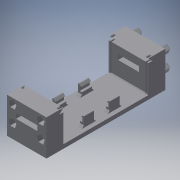
# Autodesk Inventor part: updated token 18mm
Saved by Autodesk Inventor 2018 (Build 220112000, 112)
## iProperties
Created: 2020-11-10
Part Number: updated token 18mm
Material: Generic
Document SubType Name: Modeling
Designer: Olivi
Density: 1 g/cm^3
Appearance: Default
Author: Olivi
Autodesk Inventor part; units mm, degrees
ref_plane "YZ Plane" through (0, 0, 0) normal (1, 0, 0) x (0, 1, 0)
ref_plane "XZ Plane" through (0, 0, 0) normal (0, 1, 0) x (-1, 0, 0)
ref_plane "XY Plane" through (0, 0, 0) normal (0, 0, 1) x (1, 0, 0)
sketch "Sketch1" plane through (0, 0, 0) normal (0, 0, 1) x (1, 0, 0)
  line L0 (0, 0) -> (20, 0)
  line L1 (20, 0) -> (20, 50)
  line L2 (20, 50) -> (0, 50)
  line L3 (0, 50) -> (0, 0)
  dimension "d0" = 20
  dimension "d1" = 50
  constraints: 8 end point, 2 parallel, 1 horizontal, 1 perpendicular
  measures "d0" distance of L2.end L1.end
  measures "d1" distance of L1.end L0.end
extrude "Extrusion1" add sketch "Sketch1" along normal blind 2
sketch "Sketch8" plane through (0, 0, 2) normal (0, 0, 1) x (1, 0, 0)
  line L0 (0, 0) -> (20, 0) projected
  line L1 (20, 0) -> (20, 50) projected
  line L2 (0, 0) -> (20, 0)
  line L3 (20, 0) -> (20, 8.5)
  line L4 (20, 8.5) -> (0, 8.5)
  line L5 (0, 8.5) -> (0, 0)
  dimension "d39" = 8.5
  constraints: 8 end point, 2 parallel, 1 horizontal, 1 perpendicular, 1 point on line
  measures "d39" distance of L3.end L2.end
extrude "Extrusion8" add sketch "Sketch8" along normal blind 16
sketch "Sketch9" plane through (0, 0, 0) normal (0, -1, 0) x (1, 0, 0)
  line L0 (20, 0) -> (20, 18) projected
  line L1 (0, 18) -> (20, 18) projected
  line L2 (0, 0) -> (0, 18) projected
  line L3 (4.67, 12.27) -> (15.33, 12.27)
  line L4 (15.33, 12.27) -> (15.33, 9.73)
  line L5 (15.33, 9.73) -> (4.67, 9.73)
  line L6 (4.67, 9.73) -> (4.67, 12.27)
  dimension "d42" = 4.67
  dimension "d43" = 4.67
  dimension "d45" = 2.54
  dimension "d48" = 5.73
  constraints: 8 end point, 2 parallel, 1 horizontal, 1 perpendicular
  measures "d42" distance between parallel lines of L2 L6
  measures "d43" distance between parallel lines of L0 L4
  measures "d45" distance between parallel lines of L3 L5
  measures "d48" distance between parallel lines of L1 L3
extrude "Extrusion9" cut sketch "Sketch9" against normal blind 8.5
sketch "Sketch10" plane through (0, 50, 0) normal (0, 1, 0) x (1, 0, 0)
  line L0 (0, 0) -> (20, 0) projected
  line L1 (20, -2) -> (0, -2)
  line L2 (0, -2) -> (0, 0)
  line L3 (0, 0) -> (20, 0)
  line L4 (20, 0) -> (20, -2)
  constraints: 8 end point, 2 parallel, 1 horizontal, 1 perpendicular
extrude "Extrusion10" add sketch "Sketch10" along normal blind 10
sketch "Sketch11" plane through (0, 0, 2) normal (0, 0, 1) x (1, 0, 0)
  line L0 (20, 8.5) -> (20, 60) projected
  line L1 (0, 60) -> (20, 60) projected
  line L2 (0, 60) -> (20, 60)
  line L3 (20, 60) -> (20, 51.5)
  line L4 (20, 51.5) -> (0, 51.5)
  line L5 (0, 51.5) -> (0, 60)
  point P0 (0, 0)
  dimension "d51" = 8.5
  constraints: 8 end point, 2 parallel, 1 horizontal, 1 perpendicular, 1 point on line
  measures "d51" distance of L4.end L1.start
extrude "Extrusion11" add sketch "Sketch11" along normal blind 16
sketch "Sketch12" plane through (0, 60, 0) normal (0, 1, 0) x (1, 0, 0)
  line L0 (15.33, -9.73) -> (15.33, -12.27) projected
  line L1 (4.67, -12.27) -> (4.67, -9.73) projected
  line L2 (15.33, -12.27) -> (4.67, -12.27)
  line L3 (4.67, -12.27) -> (4.67, -9.73)
  line L4 (4.67, -9.73) -> (15.33, -9.73)
  line L5 (15.33, -9.73) -> (15.33, -12.27)
  constraints: 8 end point, 2 parallel, 1 horizontal, 1 perpendicular
extrude "Extrusion12" cut sketch "Sketch12" against normal blind 8.5
sketch "Sketch13" plane through (0, 51.5, 2) normal (0, -1, 0) x (1, 0, 0)
  line L0 (20, 0) -> (0, 0) projected
  line L1 (20, 0) -> (20, 16) projected
  line L2 (0, 16) -> (20, 16) projected
  line L3 (0, 0) -> (0, 16) projected
  line L4 (0.7, 16) -> (1.3, 16)
  line L5 (1.3, 16) -> (1.3, 0)
  line L6 (1.3, 0) -> (0.7, 0)
  line L7 (0.7, 0) -> (0.7, 16)
  line L8 (19.3, 16) -> (18.7, 16)
  line L9 (18.7, 16) -> (18.7, 0)
  line L10 (18.7, 0) -> (19.3, 0)
  line L11 (19.3, 0) -> (19.3, 16)
  point P0 (0, -2)
  dimension "d63" = 0.6
  dimension "d64" = 0.7
  dimension "d65" = 0.7
  dimension "d66" = 0.6
  constraints: 16 end point, 4 parallel, 4 point on line, 2 horizontal, 2 perpendicular
  measures "d63" distance between parallel lines of L5 L7
  measures "d64" distance between parallel lines of L3 L7
  measures "d65" distance between parallel lines of L1 L11
  measures "d66" distance between parallel lines of L11 L9
extrude "Extrusion13" cut sketch "Sketch13" against normal blind 2 contours L0 L9 L2 L11 | L0 L7 L2 L5
sketch "Sketch14" plane through (0, 8.5, 2) normal (0, 1, 0) x (1, 0, 0)
  line L0 (0, 0) -> (20, 0) projected
  line L1 (0, 0) -> (0, -16) projected
  line L2 (20, -16) -> (0, -16) projected
  line L3 (20, 0) -> (20, -16) projected
  line L4 (19.3, 0) -> (18.7, 0)
  line L5 (18.7, 0) -> (18.7, -16)
  line L6 (18.7, -16) -> (19.3, -16)
  line L7 (19.3, -16) -> (19.3, 0)
  line L8 (0.7, 0) -> (1.3, 0)
  line L9 (1.3, 0) -> (1.3, -16)
  line L10 (1.3, -16) -> (0.7, -16)
  line L11 (0.7, -16) -> (0.7, 0)
  point P0 (0, 2)
  dimension "d69" = 0.7
  dimension "d70" = 0.7
  dimension "d71" = 0.6
  dimension "d72" = 0.6
  constraints: 16 end point, 4 parallel, 4 point on line, 2 horizontal, 2 perpendicular
  measures "d69" distance between parallel lines of L3 L7
  measures "d70" distance between parallel lines of L1 L11
  measures "d71" distance between parallel lines of L11 L9
  measures "d72" distance between parallel lines of L7 L5
extrude "Extrusion14" cut sketch "Sketch14" against normal blind 2 contours L0 L9 L2 L11 | L0 L7 L2 L5
sketch "Sketch15" plane through (0, 0, 0) normal (0, -1, 0) x (1, 0, 0)
  line L0 (4.67, 9.73) -> (4.67, 12.27) projected
  line L1 (4.67, 12.27) -> (15.33, 12.27) projected
  line L2 (15.33, 12.27) -> (15.33, 9.73) projected
  line L3 (1.67, 13.4183) -> (0.9284, 15.7009)
  line L4 (0.9284, 15.7009) -> (2.87, 17.1116)
  line L5 (2.87, 17.1116) -> (4.8116, 15.7009)
  line L6 (4.8116, 15.7009) -> (4.07, 13.4183)
  line L7 (4.07, 13.4183) -> (1.67, 13.4183)
  line L8 (15.93, 13.4183) -> (15.1884, 15.7009)
  line L9 (15.1884, 15.7009) -> (17.13, 17.1116)
  line L10 (17.13, 17.1116) -> (19.0716, 15.7009)
  line L11 (19.0716, 15.7009) -> (18.33, 13.4183)
  line L12 (18.33, 13.4183) -> (15.93, 13.4183)
  line L13 (1.67, 5.2783) -> (0.9284, 7.5609)
  line L14 (0.9284, 7.5609) -> (2.87, 8.9716)
  line L15 (2.87, 8.9716) -> (4.8116, 7.5609)
  line L16 (4.8116, 7.5609) -> (4.07, 5.2783)
  line L17 (4.07, 5.2783) -> (1.67, 5.2783)
  line L18 (15.93, 5.2783) -> (15.1884, 7.5609)
  line L19 (15.1884, 7.5609) -> (17.13, 8.9716)
  line L20 (17.13, 8.9716) -> (19.0716, 7.5609)
  line L21 (19.0716, 7.5609) -> (18.33, 5.2783)
  line L22 (18.33, 5.2783) -> (15.93, 5.2783)
  point P0 (2.87, 15.07)
  point P1 (17.13, 15.07)
  point P2 (2.87, 6.93)
  point P3 (17.13, 6.93)
  dimension "d95" = 2.4
  dimension "d96" = 1.8
  dimension "d97" = 2.8
  dimension "d98" = 2.4
  dimension "d99" = 1.8
  dimension "d100" = 2.8
  dimension "d101" = 2.4
  dimension "d102" = 2.4
  dimension "d184" = 8.14
  constraints: 40 end point, 2 vertical alignment, 1 horizontal alignment, 44 other
  measures "d95" distance of L6.end L3.start
  measures "d96" distance from line of L0 point (2.87, 15.07)
  measures "d97" distance from line of point (2.87, 15.07) L1
  measures "d98" distance of L11.end L8.start
  measures "d99" distance from line of L2 point (17.13, 15.07)
  measures "d100" distance from line of point (17.13, 15.07) L1
  measures "d101" distance of L16.end L13.start
  measures "d102" distance of L21.end L18.start
  measures "d184" distance of point (2.87, 6.93) point (2.87, 15.07)
extrude "Extrusion15" cut sketch "Sketch15" against normal blind 4
sketch "Sketch16" plane through (0, 60, 0) normal (0, 1, 0) x (1, 0, 0)
  line L0 (15.3906, -15.6352) -> (16.055, -13.5904)
  line L1 (16.055, -13.5904) -> (18.205, -13.5904)
  line L2 (18.205, -13.5904) -> (18.8694, -15.6352)
  line L3 (18.8694, -15.6352) -> (17.13, -16.8989)
  line L4 (17.13, -16.8989) -> (15.3906, -15.6352)
  line L5 (4.6094, -15.6352) -> (2.87, -16.8989)
  line L6 (2.87, -16.8989) -> (1.1306, -15.6352)
  line L7 (1.1306, -15.6352) -> (1.795, -13.5904)
  line L8 (1.795, -13.5904) -> (3.945, -13.5904)
  line L9 (3.945, -13.5904) -> (4.6094, -15.6352)
  line L10 (4.6094, -7.4952) -> (2.87, -8.7589)
  line L11 (2.87, -8.7589) -> (1.1306, -7.4952)
  line L12 (1.1306, -7.4952) -> (1.795, -5.4504)
  line L13 (1.795, -5.4504) -> (3.945, -5.4504)
  line L14 (3.945, -5.4504) -> (4.6094, -7.4952)
  line L15 (16.055, -5.4504) -> (18.205, -5.4504)
  line L16 (18.205, -5.4504) -> (18.8694, -7.4952)
  line L17 (18.8694, -7.4952) -> (17.13, -8.7589)
  line L18 (17.13, -8.7589) -> (15.3906, -7.4952)
  line L19 (15.3906, -7.4952) -> (16.055, -5.4504)
  line L20 (20, -18) -> (0, -18) projected
  line L21 (20, 0) -> (20, -18) projected
  line L22 (15.33, -12.27) -> (4.67, -12.27) projected
  line L23 (4.67, -9.73) -> (15.33, -9.73) projected
  line L24 (15.33, -12.27) -> (4.67, -12.27)
  line L25 (4.67, -12.27) -> (4.67, -9.73)
  line L26 (4.67, -9.73) -> (15.33, -9.73)
  line L27 (15.33, -9.73) -> (15.33, -12.27)
  point P0 (17.13, -15.07)
  point P1 (2.87, -15.07)
  point P2 (2.87, -6.93)
  point P3 (17.13, -6.93)
  dimension "d141" = 2.15
  dimension "d142" = 2.15
  dimension "d143" = 2.15
  dimension "d144" = 2.15
  dimension "d185" = 8.14
  dimension "d186" = 2.93
  dimension "d187" = 2.87
  dimension "d191" = 14.26
  constraints: 48 end point, 2 horizontal alignment, 2 parallel, 2 vertical alignment, 1 horizontal, 1 perpendicular, 44 other
  measures "d141" distance of L0.end L1.end
  measures "d142" distance of L7.end L8.end
  measures "d143" distance of L12.end L13.end
  measures "d144" distance of L15.start L15.end
  measures "d185" distance of point (17.13, -6.93) point (17.13, -15.07)
  measures "d186" distance from line of L20 point (17.13, -15.07)
  measures "d187" distance from line of L21 point (17.13, -15.07)
  measures "d191" distance of point (2.87, -15.07) point (17.13, -15.07)
extrude "Extrusion16" add sketch "Sketch16" along normal blind 4 contours L0 L1 L2 L3 L4 | L5 L6 L7 L8 L9 | L10 L11 L12 L13 L14 | L15 L16 L17 L18 L19
chamfer "Chamfer4" distance 0.5 angle 45 20 edges at (3.7397, 64, 16.267) (2.0003, 64, 16.267) (4.2772, 64, 14.6128) (2.87, 64, 13.5904) (1.4628, 64, 14.6128) (17.9997, 64, 16.267) (16.2603, 64, 16.267) (3.7397, 64, 8.127) (2.0003, 64, 8.127) (1.4628, 64, 6.4728) (2.87, 64, 5.4504) (4.2772, 64, 6.4728) (17.9997, 64, 8.127) (16.2603, 64, 8.127) (15.7228, 64, 6.4728) (17.13, 64, 5.4504) (18.5372, 64, 6.4728) (18.5372, 64, 14.6128) (17.13, 64, 13.5904) (15.7228, 64, 14.6128)
sketch "Sketch20" plane through (0, 0, 2) normal (0, 0, 1) x (1, 0, 0)
  line L0 (18.7, 51.5) -> (1.3, 51.5) projected
  line L1 (0, 8.5) -> (0, 51.5) projected
  line L2 (2, 39) -> (18, 39)
  line L3 (18, 39) -> (18, 21)
  line L4 (18, 21) -> (2, 21)
  line L5 (2, 21) -> (2, 39)
  point P0 (0, 0)
  dimension "d148" = 16
  dimension "d149" = 18
  dimension "d150" = 2
  dimension "d151" = 12.5
  constraints: 8 end point, 2 parallel, 1 horizontal, 1 perpendicular
  measures "d148" distance of L3.end L4.end
  measures "d149" distance of L2.end L3.end
  measures "d150" distance between parallel lines of L1 L5
  measures "d151" distance between parallel lines of L0 L2
extrude "Extrusion19" add sketch "Sketch20" along normal blind 5
sketch "Sketch21" plane through (2, 21, 2) normal (0, -1, 0) x (1, 0, 0)
  line L0 (16, 0) -> (0, 0) projected
  line L1 (0, 5) -> (16, 5) projected
  line L2 (0, 0) -> (0, 5) projected
  line L3 (0, 0) -> (2, 0)
  line L4 (2, 0) -> (2, 2)
  line L5 (2, 2) -> (0, 2)
  line L6 (0, 2) -> (0, 0)
  line L7 (16, 0) -> (14, 0)
  line L8 (14, 0) -> (14, 2)
  line L9 (14, 2) -> (16, 2)
  line L10 (16, 2) -> (16, 0)
  line L11 (0, 2) -> (0.8, 2)
  line L12 (0.8, 2) -> (0.8, 4)
  line L13 (0.8, 4) -> (0, 4)
  line L14 (0, 4) -> (0, 2)
  line L15 (16, 2) -> (15.2, 2)
  line L16 (15.2, 2) -> (15.2, 4)
  line L17 (15.2, 4) -> (16, 4)
  line L18 (16, 4) -> (16, 2)
  line L19 (0, 5) -> (1.5, 5)
  line L20 (1.5, 5) -> (1.5, 4)
  line L21 (1.5, 4) -> (0, 4)
  line L22 (0, 4) -> (0, 5)
  line L23 (16, 4) -> (14.5, 4)
  line L24 (14.5, 4) -> (14.5, 5)
  line L25 (14.5, 5) -> (16, 5)
  line L26 (16, 5) -> (16, 4)
  point P0 (-2, -2)
  dimension "d154" = 2
  dimension "d155" = 2
  dimension "d156" = 2
  dimension "d157" = 2
  dimension "d158" = 0.8
  dimension "d159" = 2
  dimension "d160" = 0.8
  dimension "d161" = 2
  dimension "d162" = 1.5
  dimension "d163" = 1.5
  constraints: 48 end point, 12 parallel, 6 horizontal, 6 perpendicular, 1 point on line
  measures "d154" distance of L5.end L4.end
  measures "d155" distance of L4.end L3.end
  measures "d156" distance of L8.end L9.end
  measures "d157" distance of L7.end L8.end
  measures "d158" distance of L13.end L12.end
  measures "d159" distance of L12.end L11.end
  measures "d160" distance of L16.end L17.end
  measures "d161" distance of L15.end L16.end
  measures "d162" distance of L20.end L21.end
  measures "d163" distance of L24.end L25.end
extrude "Extrusion20" cut sketch "Sketch21" against normal blind 18 contours L0 L4 L5 L12 L21 L20 L1 L24 L23 L16 L9 L8
sketch "Sketch22" plane through (2, 21, 2) normal (-1, 0, 0) x (0, 0, 1)
  line L0 (0, 0) -> (5, 0) projected
  line L1 (5, 0) -> (5, 18) projected
  line L2 (0, 18) -> (0, 0) projected
  line L3 (5, 13) -> (0, 13)
  line L4 (0, 13) -> (0, 5)
  line L5 (0, 5) -> (5, 5)
  line L6 (5, 5) -> (5, 13)
  point P0 (-2, -21)
  dimension "d169" = 8
  dimension "d170" = 5
  constraints: 8 end point, 2 parallel, 2 point on line, 1 horizontal, 1 perpendicular
  measures "d169" distance of L4.end L3.end
  measures "d170" distance between parallel lines of L0 L5
extrude "Extrusion21" cut sketch "Sketch22" against normal blind 18 contours L2 L3 L1 L5
sketch "Sketch23" plane through (20, 0, 18) normal (1, 0, 0) x (0, 0, -1)
  line L0 (16, 51.5) -> (0, 51.5) projected
  line L1 (0, 8.5) -> (2, 8.5)
  line L2 (16, 8.5) -> (0, 8.5) projected
  line L3 (2, 8.5) -> (2, 6.5)
  line L4 (2, 6.5) -> (0, 8.5)
  line L5 (0, 51.5) -> (2, 51.5)
  line L6 (2, 51.5) -> (2, 53.5)
  line L7 (0, 51.5) -> (16, 51.5) projected
  line L8 (2, 53.5) -> (0, 51.5)
  dimension "d173" = 2
  dimension "d174" = 2
  dimension "d175" = 2
  constraints: 12 end point, 4 point on line, 1 perpendicular
  measures "d173" distance of L1.start L1.end
  measures "d174" distance of L1.end L3.end
  measures "d175" distance of L5.end L6.end
extrude "Extrusion22" cut sketch "Sketch23" against normal through all
chamfer "Chamfer6" distance 1 angle 45 4 edges at (3.5, 23.5, 7) (3.5, 36.5, 7) (16.5, 23.5, 7) (16.5, 36.5, 7)
chamfer "Chamfer7" distance 1 angle 45 8 edges at (3, 34, 2) (17, 34, 2) (17, 21, 2) (3, 26, 2) (17, 39, 2) (17, 26, 2) (3, 39, 2) (3, 21, 2)
chamfer "Chamfer8" distance 0.25 angle 45 8 edges at (18.7, 7.5, 18) (19.3, 7.5, 18) (0.7, 7.5, 18) (1.3, 7.5, 18) (18.7, 52.5, 18) (19.3, 52.5, 18) (0.7, 52.5, 18) (1.3, 52.5, 18)
chamfer "Chamfer9" distance 0.5 angle 45 2 edges at (10, 8.5, 2) (10, 51.5, 2)
body "Solid1"
